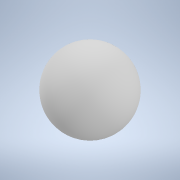
# Autodesk Inventor part: 25_Sfere
Saved by Autodesk Inventor 2020.2 (Build 242310000, 310)
## iProperties
Created: 2019-11-29
Part Number: 25_Sfere
Material: Geomag
Document SubType Name: Modeling
Designer: socci
Density: 8.391 g/cm^3
Appearance: Default
Mass: 8.99961 g
Surface Area: 5.06707 cm^2
Volume: 1.07253 cm^3
Author: socci
Autodesk Inventor part; units mm, degrees
ref_plane "YZ Plane" through (0, 0, 0) normal (1, 0, 0) x (0, 1, 0)
ref_plane "XZ Plane" through (0, 0, 0) normal (0, 1, 0) x (-1, 0, 0)
ref_plane "XY Plane" through (0, 0, 0) normal (0, 0, 1) x (1, 0, 0)
sketch "Schizzo1" plane through (0, 0, 0) normal (0, 1, 0) x (-1, 0, 0)
  arc A0 (-6.35, 0) -> (6.35, 0) centre (0, 0) ccw
  line L0 (-6.35, 0) -> (6.35, 0)
  line L1 (0, 0) -> (10, 0) construction
  line L2 (0, 0) -> (5, 0) construction
  line L3 (3.9144, -5) -> (3.9144, 0)
  line L4 (-3.9144, -5) -> (-3.9144, 0)
  dimension "d6" = 12.7
  constraints: 10 end point, 3 horizontal, 3 point on circle, 2 perpendicular, 2 point on line, 1 centre point
  measures "d6" distance of L0.start L0.end
revolve "Rivoluzione1" add sketch "Schizzo1" angle 360 about axis through (6.35, 0, 0) along (-1, 0, 0)
